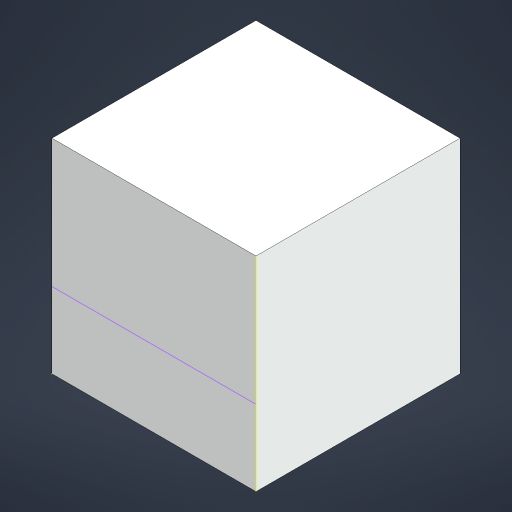
# Autodesk Inventor part: skeleton
Saved by Autodesk Inventor 2023.1 (Build 271208000, 208)
## iProperties
Created: 2022-11-09
Part Number: skeleton
Material: Generic
Document SubType Name: Modeling
Designer: awelt
Mass: 131097 g
Surface Area: 15483.8 cm^2
Volume: 131097 cm^3
Density: 1 g/cm^3
Appearance: Default
RuleStatus: InUse
BeforeDocSave0: file://C:\Users\awelt\Documents\Inventor\iLogic_Rules\BoundingStore
DocClose0: file://C:\Users\awelt\Documents\Inventor\iLogic_Rules\BoundingStore
Author: awelt
BoundingBL1: 20
BoundingBL2: 20
BoundingBL3: 20
BoundingCF: 4.63
Autodesk Inventor part; units mm, degrees
ref_plane "YZ Plane" through (0, 0, 0) normal (1, 0, 0) x (0, 1, 0)
ref_plane "XZ Plane" through (0, 0, 0) normal (0, 1, 0) x (-1, 0, 0)
ref_plane "XY Plane" through (0, 0, 0) normal (0, 0, 1) x (1, 0, 0)
sketch "Sketch2" plane through (0, 0, 0) normal (0, 1, 0) x (-1, 0, 0)
  line L0 (0, 0) -> (-508, 0)
  line L1 (-508, 0) -> (-508, -508)
  line L2 (-508, -508) -> (0, -508)
  line L3 (0, -508) -> (0, 0)
  dimension "d3" = 508
  dimension "d4" = 508
  constraints: 8 end point, 2 parallel, 1 horizontal, 1 perpendicular
  measures "d3" distance of L2.end L1.end
  measures "d4" distance of L1.end L0.end
extrude "Extrusion1" add sketch "Sketch2" along normal blind 508
sketch "Sketch3" plane through (0, 0, 0) normal (0, 0, 1) x (1, 0, 0)
  line L0 (0, 188.3898) -> (508, 188.3898)
  line L1 (508, 0) -> (508, 508) projected
  point P0 (0, 0)
  constraints: 2 end point, 1 horizontal, 1 point on line
body "Solid1"
